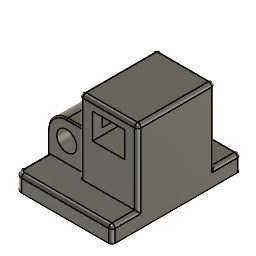
Front Dozer Seat (Autodesk Fusion 360 design; units mm, degrees)
part number: 2026-03-22-23-02-17-136
Autodesk Fusion 360 part; units mm, degrees
sketch "Sketch1" plane through (0, 0, 0) normal (0, 0, 1) x (1, 0, 0)
  line L0 (19.05, -25.4) -> (-19.05, -25.4)
  line L1 (-19.05, -25.4) -> (-19.05, 25.4)
  line L2 (-19.05, 25.4) -> (19.05, 25.4)
  line L3 (19.05, 25.4) -> (19.05, -25.4)
  line L4 (19.05, -25.4) -> (-19.05, 25.4) construction
  line L5 (-19.05, -25.4) -> (19.05, 25.4) construction
  dimension "d1" = 38.1
  dimension "d2" = 50.8
  constraint horizontal L0
  constraint perpendicular L0 L1
  constraint parallel L0 L2
  constraint parallel L1 L3
  constraint coincident L4 origin
  constraint coincident L5 origin
  measures "d1" distance of L1.end L2.end
  measures "d2" distance of L0.end L1.end
extrude "Extrude1" add sketch "Sketch1" along normal blind 6.35
sketch "Sketch2" plane through (0, 0, 6.35) normal (0, 0, 1) x (-1, 0, 0)
  line L0 (-19.05, -25.4) -> (19.05, -25.4)
  line L1 (19.05, -25.4) -> (19.05, 25.4)
  line L2 (19.05, 25.4) -> (-19.05, 25.4)
  line L3 (-19.05, 25.4) -> (-19.05, -25.4)
  line L4 (19.05, -12.7) -> (3.81, -12.7)
  line L5 (3.81, -12.7) -> (3.81, 12.7)
  line L6 (3.81, 12.7) -> (19.05, 12.7)
  line L7 (19.05, 12.7) -> (19.05, -12.7)
  line L8 (-19.05, -15.24) -> (3.81, -15.24)
  line L9 (3.81, -15.24) -> (3.81, 15.24)
  line L10 (3.81, 15.24) -> (-19.05, 15.24)
  line L11 (-19.05, 15.24) -> (-19.05, -15.24)
  dimension "d5" = 15.24
  dimension "d6" = 25.4
  dimension "d7" = 12.7
  dimension "d9" = 10.16
  dimension "d14" = 10.16
  constraint horizontal L4
  constraint vertical L5
  constraint horizontal L6
  constraint vertical L7
  constraint coincident L1 L4.start
  constraint horizontal L8
  constraint vertical L9
  constraint horizontal L10
  constraint vertical L11
  constraint coincident L3 L8.start
  constraint collinear L5 L9
  measures "d5" distance of L7 L9
  measures "d6" distance of L4 L6
  measures "d7" distance of L0 L4
  measures "d9" distance of L0 L8
  measures "d14" distance of L2 L10
extrude "Extrude2" add sketch "Sketch2" along normal blind 15.24 contours L1 L4 L5 L6 L7 L9
extrude "Extrude3" add sketch "Sketch2" along normal blind 29.21 contours L3 L5 L8 L9 L10 L11
sketch "Sketch3" plane through (0, -12.7, 0) normal (0, -1, 0) x (1, 0, 0)
  line L0 (-19.05, 6.35) -> (-3.81, 6.35)
  line L1 (-3.81, 6.35) -> (-3.81, 21.59)
  line L2 (-3.81, 21.59) -> (-19.05, 21.59)
  line L3 (-19.05, 21.59) -> (-19.05, 6.35)
  circle A0 centre (-11.43, 13.97) radius 3.937
  dimension "d15" = 7.874
  dimension "d16" = 7.62
  dimension "d17" = 7.62
  measures "d15" diameter of A0
  measures "d16" distance of L2 A0.centre
  measures "d17" distance of L3 A0.centre
extrude "Extrude4" cut sketch "Sketch3" against normal through all contours A0
fillet "Fillet1" radius 2.54 2 edges at (-19.05, -25.4, 3.175) (-19.05, 25.4, 3.175)
fillet "Fillet2" radius 1.27 6 edges at (1.27, 25.4, 6.35) (-18.3061, 24.6561, 6.35) (-19.05, 17.78, 6.35) (-19.05, -17.78, 6.35) (-18.3061, -24.6561, 6.35) (1.27, -25.4, 6.35)
fillet "Fillet3" radius 7.62 1 edges at (-19.05, 0, 21.59)
fillet "Fillet4" radius 1.27 14 edges at (-3.81, 15.24, 20.955) (7.62, 15.24, 35.56) (-3.81, 0, 35.56) (7.62, -15.24, 35.56) (-3.81, -15.24, 20.955) (19.05, 0, 35.56) (19.05, -15.24, 20.955) (19.05, 15.24, 20.955) (19.05, -25.4, 2.54) (19.05, -25.028, 5.978) (19.05, -19.685, 6.35) (19.05, 19.685, 6.35) (19.05, 25.028, 5.978) (19.05, 25.4, 2.54)
fillet "Fillet5" radius 0.508 6 edges at (-7.62, 12.7, 21.59) (-16.8182, 12.7, 19.3582) (-19.05, 12.7, 9.525) (-19.05, -12.7, 9.525) (-16.8182, -12.7, 19.3582) (-7.62, -12.7, 21.59)
sketch "Sketch4" plane through (0, 15.24, 0) normal (0, 1, 0) x (-1, 0, 0)
  line L0 (2.54, 6.35) -> (2.54, 34.29)
  line L1 (2.54, 34.29) -> (-17.78, 34.29)
  line L2 (-17.78, 34.29) -> (-17.78, 6.35)
  line L3 (-17.78, 6.35) -> (2.54, 6.35)
  line L4 (-13.97, 31.75) -> (-1.27, 31.75)
  line L5 (-1.27, 31.75) -> (-1.27, 21.59)
  line L6 (-1.27, 21.59) -> (-13.97, 21.59)
  line L7 (-13.97, 21.59) -> (-13.97, 31.75)
  dimension "d29" = 3.81
  dimension "d30" = 3.81
  dimension "d31" = 2.54
  dimension "d32" = 10.16
  constraint horizontal L4
  constraint vertical L5
  constraint horizontal L6
  constraint vertical L7
  measures "d29" distance of L2 L7
  measures "d30" distance of L0 L5
  measures "d31" distance of L1 L4
  measures "d32" distance of L4 L6
extrude "Extrude5" cut sketch "Sketch4" against normal through all contours L4 L5 L6 L7
sketch "Sketch5" plane through (-3.81, 0, 0) normal (-1, 0, 0) x (0, -1, 0)
  line L0 (13.97, 6.35) -> (13.97, 34.29)
  line L1 (13.97, 34.29) -> (-13.97, 34.29)
  line L2 (-13.97, 34.29) -> (-13.97, 6.35)
  line L3 (-13.97, 6.35) -> (-12.7, 6.35)
  line L4 (-12.7, 6.35) -> (-12.7, 21.082)
  arc A0 (-12.192, 21.59) -> (-12.7, 21.082) centre (-12.192, 21.082) ccw
  line L5 (-12.192, 21.59) -> (12.192, 21.59)
  arc A1 (12.7, 21.082) -> (12.192, 21.59) centre (12.192, 21.082) ccw
  line L6 (12.7, 21.082) -> (12.7, 6.35)
  line L7 (12.7, 6.35) -> (13.97, 6.35)
  line L8 (-11.43, 33.02) -> (11.43, 33.02)
  line L9 (11.43, 33.02) -> (11.43, 24.2438)
  line L10 (11.43, 24.2438) -> (-11.43, 24.2438)
  line L11 (-11.43, 24.2438) -> (-11.43, 33.02)
  constraint horizontal L8
  constraint vertical L9
  constraint horizontal L10
  constraint vertical L11
extrude "Extrude6" cut sketch "Sketch5" against normal up to surface (17.78 mm away) contours L8 L9 L10 L11
sketch "Sketch6" plane through (0, 0, 0) normal (0, 0, -1) x (1, 0, 0)
  arc A0 (19.05, 24.13) -> (17.78, 25.4) centre (17.78, 24.13) ccw
  line L0 (17.78, 25.4) -> (-16.51, 25.4)
  arc A1 (-16.51, 25.4) -> (-19.05, 22.86) centre (-16.51, 22.86) ccw
  line L1 (-19.05, 22.86) -> (-19.05, -22.86)
  arc A2 (-19.05, -22.86) -> (-16.51, -25.4) centre (-16.51, -22.86) ccw
  line L2 (-16.51, -25.4) -> (17.78, -25.4)
  arc A3 (17.78, -25.4) -> (19.05, -24.13) centre (17.78, -24.13) ccw
  line L3 (19.05, -24.13) -> (19.05, 24.13)
  circle A4 centre (0, 0) radius 3.5
  dimension "d36" = 7
  constraint coincident A4.centre origin
  measures "d36" diameter of A4
extrude "Extrude7" cut sketch "Sketch6" against normal blind 2 contours A4
